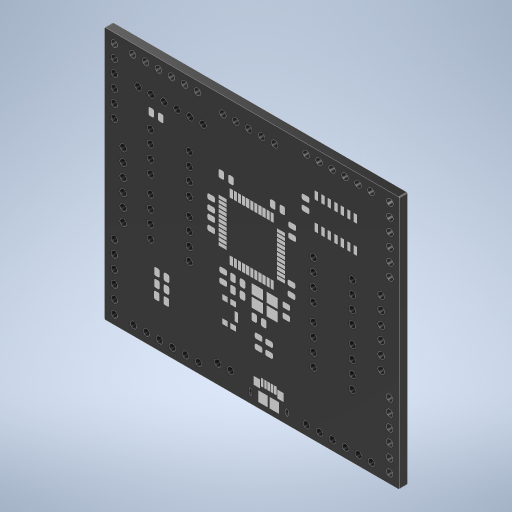
# Autodesk Inventor part: Birty.kicad_pcb
Saved by Autodesk Inventor 2023 (Build 270158000, 158)
## iProperties
Created: 2022-05-19
Part Number: Birty.kicad_pcb
Material: Generic
Document SubType Name: Modeling
Designer: Jack2bs
Density: 1 g/cm^3
Appearance: Glossy - Black
Author: Jack2bs
Autodesk Inventor part; units mm, degrees
(part 1 of 3)
ref_plane "YZ Plane" through (0, 0, 0) normal (1, 0, 0) x (0, 1, 0)
ref_plane "XZ Plane" through (0, 0, 0) normal (0, 1, 0) x (-1, 0, 0)
ref_plane "XY Plane" through (0, 0, 0) normal (0, 0, 1) x (1, 0, 0)
sketch "Sketch1" plane through (0, 0, 0) normal (0, 0, 1) x (1, 0, 0)
  line L0 (84.8868, -104.3178) -> (84.8868, -153.6446)
  arc A0 (84.8868, -153.6446) -> (85.0138, -153.7716) centre (85.0138, -153.6446) ccw
  line L1 (85.0138, -153.7716) -> (142.4432, -153.7716)
  arc A1 (142.4432, -153.7716) -> (142.5702, -153.6446) centre (142.4432, -153.6446) ccw
  line L2 (142.5702, -153.6446) -> (142.5702, -104.3178)
  arc A2 (142.5702, -104.3178) -> (142.4432, -104.1908) centre (142.4432, -104.3178) ccw
  line L3 (142.4432, -104.1908) -> (85.0138, -104.1908)
  arc A3 (85.0138, -104.1908) -> (84.8868, -104.3178) centre (85.0138, -104.3178) ccw
  line L4 (120.8178, -151.3204) -> (120.8178, -152.1204)
  arc A4 (120.3678, -152.1204) -> (120.8178, -152.1204) centre (120.5928, -152.1204) ccw
  line L5 (120.3678, -152.1204) -> (120.3678, -151.3204)
  arc A5 (120.8178, -151.3204) -> (120.3678, -151.3204) centre (120.5928, -151.3204) ccw
  line L6 (113.2178, -152.1204) -> (113.2178, -151.3204)
  arc A6 (113.6678, -151.3204) -> (113.2178, -151.3204) centre (113.4428, -151.3204) ccw
  line L7 (113.6678, -151.3204) -> (113.6678, -152.1204)
  arc A7 (113.2178, -152.1204) -> (113.6678, -152.1204) centre (113.4428, -152.1204) ccw
  circle A8 centre (103.0766, -106.067) radius 0.635
  circle A9 centre (100.5366, -106.067) radius 0.635
  circle A10 centre (92.9166, -106.067) radius 0.635
  circle A11 centre (95.4566, -106.067) radius 0.635
  circle A12 centre (90.3766, -106.067) radius 0.635
  circle A13 centre (97.9966, -106.067) radius 0.635
  circle A14 centre (137.0364, -106.0162) radius 0.635
  circle A15 centre (134.4964, -106.0162) radius 0.635
  circle A16 centre (126.8764, -106.0162) radius 0.635
  circle A17 centre (129.4164, -106.0162) radius 0.635
  circle A18 centre (124.3364, -106.0162) radius 0.635
  circle A19 centre (131.9564, -106.0162) radius 0.635
  circle A20 centre (88.519, -122.8344) radius 0.6475
  circle A21 centre (88.519, -125.3744) radius 0.6475
  circle A22 centre (88.519, -127.9144) radius 0.6475
  circle A23 centre (88.519, -130.4544) radius 0.6475
  circle A24 centre (88.519, -132.9944) radius 0.6475
  circle A25 centre (88.519, -135.5344) radius 0.6475
  circle A26 centre (139.0396, -135.3312) radius 0.6475
  circle A27 centre (139.0396, -132.7912) radius 0.6475
  circle A28 centre (139.0396, -130.2512) radius 0.6475
  circle A29 centre (139.0396, -127.7112) radius 0.6475
  circle A30 centre (139.0396, -125.1712) radius 0.6475
  circle A31 centre (139.0396, -122.6312) radius 0.6475
  circle A32 centre (86.763, -106.067) radius 0.635
  circle A33 centre (86.763, -108.607) radius 0.635
  circle A34 centre (86.763, -116.227) radius 0.635
  circle A35 centre (86.763, -113.687) radius 0.635
  circle A36 centre (86.763, -118.767) radius 0.635
  circle A37 centre (86.763, -111.147) radius 0.635
  circle A38 centre (118.1862, -107.3658) radius 0.635
  circle A39 centre (113.1062, -107.3658) radius 0.635
  circle A40 centre (108.0262, -107.3658) radius 0.635
  circle A41 centre (110.5662, -107.3658) radius 0.635
  circle A42 centre (115.6462, -107.3658) radius 0.635
  circle A43 centre (86.763, -139.2648) radius 0.635
  circle A44 centre (86.763, -141.8048) radius 0.635
  circle A45 centre (86.763, -149.4248) radius 0.635
  circle A46 centre (86.763, -146.8848) radius 0.635
  circle A47 centre (86.763, -151.9648) radius 0.635
  circle A48 centre (86.763, -144.3448) radius 0.635
  circle A49 centre (107.0102, -150.1394) radius 0.6475
  circle A50 centre (109.5502, -150.1394) radius 0.6475
  circle A51 centre (140.7448, -118.6722) radius 0.635
  circle A52 centre (140.7448, -116.1322) radius 0.635
  circle A53 centre (140.7448, -108.5122) radius 0.635
  circle A54 centre (140.7448, -111.0522) radius 0.635
  circle A55 centre (140.7448, -105.9722) radius 0.635
  circle A56 centre (140.7448, -113.5922) radius 0.635
  circle A57 centre (101.5966, -111.0776) radius 0.635
  circle A58 centre (91.4366, -111.0776) radius 0.635
  circle A59 centre (93.9766, -111.0776) radius 0.635
  circle A60 centre (96.5166, -111.0776) radius 0.635
  circle A61 centre (104.1366, -111.0776) radius 0.635
  circle A62 centre (99.0566, -111.0776) radius 0.635
  circle A63 centre (140.694, -151.8954) radius 0.635
  circle A64 centre (140.694, -149.3554) radius 0.635
  circle A65 centre (140.694, -141.7354) radius 0.635
  circle A66 centre (140.694, -144.2754) radius 0.635
  circle A67 centre (140.694, -139.1954) radius 0.635
  circle A68 centre (140.694, -146.8154) radius 0.635
  circle A69 centre (90.5476, -151.8954) radius 0.635
  circle A70 centre (93.0876, -151.8954) radius 0.635
  circle A71 centre (100.7076, -151.8954) radius 0.635
  circle A72 centre (98.1676, -151.8954) radius 0.635
  circle A73 centre (103.2476, -151.8954) radius 0.635
  circle A74 centre (95.6276, -151.8954) radius 0.635
  circle A75 centre (124.4058, -151.8954) radius 0.635
  circle A76 centre (126.9458, -151.8954) radius 0.635
  circle A77 centre (134.5658, -151.8954) radius 0.635
  circle A78 centre (132.0258, -151.8954) radius 0.635
  circle A79 centre (137.1058, -151.8954) radius 0.635
  circle A80 centre (129.4858, -151.8954) radius 0.635
  circle A81 centre (93.853, -124.6632) radius 0.635
  circle A82 centre (93.853, -122.1232) radius 0.635
  circle A83 centre (93.853, -117.0432) radius 0.635
  circle A84 centre (93.853, -119.5832) radius 0.635
  circle A85 centre (101.473, -119.5832) radius 0.635
  circle A86 centre (101.473, -117.0432) radius 0.635
  circle A87 centre (101.473, -124.6632) radius 0.635
  circle A88 centre (101.473, -122.1232) radius 0.635
  circle A89 centre (133.4008, -133.8072) radius 0.635
  circle A90 centre (133.4008, -136.3472) radius 0.635
  circle A91 centre (133.4008, -141.4272) radius 0.635
  circle A92 centre (133.4008, -138.8872) radius 0.635
  circle A93 centre (125.7808, -138.8872) radius 0.635
  circle A94 centre (125.7808, -141.4272) radius 0.635
  circle A95 centre (125.7808, -133.8072) radius 0.635
  circle A96 centre (125.7808, -136.3472) radius 0.635
  circle A97 centre (93.853, -135.6868) radius 0.635
  circle A98 centre (93.853, -133.1468) radius 0.635
  circle A99 centre (93.853, -128.0668) radius 0.635
  circle A100 centre (93.853, -130.6068) radius 0.635
  circle A101 centre (101.473, -130.6068) radius 0.635
  circle A102 centre (101.473, -128.0668) radius 0.635
  circle A103 centre (101.473, -135.6868) radius 0.635
  circle A104 centre (101.473, -133.1468) radius 0.635
  circle A105 centre (133.3754, -122.809) radius 0.635
  circle A106 centre (133.3754, -125.349) radius 0.635
  circle A107 centre (133.3754, -130.429) radius 0.635
  circle A108 centre (133.3754, -127.889) radius 0.635
  circle A109 centre (125.7554, -127.889) radius 0.635
  circle A110 centre (125.7554, -130.429) radius 0.635
  circle A111 centre (125.7554, -122.809) radius 0.635
  circle A112 centre (125.7554, -125.349) radius 0.635
  constraints: 113 centre point, 16 end point, 16 point on circle
extrude "Birty.kicad_pcb_Outline" add sketch "Sketch1" along normal blind 1.6
sketch "Sketch2" plane through (0, 0, 1.6) normal (0, 0, 1) x (1, 0, 0)
  line L0 (116.7679, -152.6705) -> (115.0178, -152.6705)
  line L1 (115.0178, -152.6705) -> (115.0178, -150.7703)
  line L2 (115.0178, -150.7703) -> (116.7679, -150.7703)
  line L3 (116.7679, -150.7703) -> (116.7679, -152.6705)
  line L4 (119.0178, -152.6705) -> (117.2677, -152.6705)
  line L5 (117.2677, -152.6705) -> (117.2677, -150.7703)
  line L6 (117.2677, -150.7703) -> (119.0178, -150.7703)
  line L7 (119.0178, -150.7703) -> (119.0178, -152.6705)
  line L8 (115.2728, -150.2153) -> (114.1227, -150.2153)
  line L9 (114.1227, -150.2153) -> (114.1227, -148.7655)
  line L10 (114.1227, -148.7655) -> (115.2728, -148.7655)
  line L11 (115.2728, -148.7655) -> (115.2728, -150.2153)
  line L12 (119.9129, -150.2153) -> (118.7628, -150.2153)
  line L13 (118.7628, -150.2153) -> (118.7628, -148.7655)
  line L14 (118.7628, -148.7655) -> (119.9129, -148.7655)
  line L15 (119.9129, -148.7655) -> (119.9129, -150.2153)
  line L16 (117.2177, -149.7703) -> (116.8179, -149.7703)
  line L17 (116.8179, -149.7703) -> (116.8179, -148.3703)
  line L18 (116.8179, -148.3703) -> (117.2177, -148.3703)
  line L19 (117.2177, -148.3703) -> (117.2177, -149.7703)
  line L20 (117.8677, -149.7703) -> (117.4679, -149.7703)
  line L21 (117.4679, -149.7703) -> (117.4679, -148.3703)
  line L22 (117.4679, -148.3703) -> (117.8677, -148.3703)
  line L23 (117.8677, -148.3703) -> (117.8677, -149.7703)
  line L24 (118.5179, -149.7703) -> (118.1179, -149.7703)
  line L25 (118.1179, -149.7703) -> (118.1179, -148.3703)
  line L26 (118.1179, -148.3703) -> (118.5179, -148.3703)
  line L27 (118.5179, -148.3703) -> (118.5179, -149.7703)
  line L28 (115.9177, -149.7703) -> (115.5177, -149.7703)
  line L29 (115.5177, -149.7703) -> (115.5177, -148.3703)
  line L30 (115.5177, -148.3703) -> (115.9177, -148.3703)
  line L31 (115.9177, -148.3703) -> (115.9177, -149.7703)
  line L32 (116.5677, -149.7703) -> (116.1679, -149.7703)
  line L33 (116.1679, -149.7703) -> (116.1679, -148.3703)
  line L34 (116.1679, -148.3703) -> (116.5677, -148.3703)
  line L35 (116.5677, -148.3703) -> (116.5677, -149.7703)
  line L36 (97.2663, -143.9832) -> (97.312, -143.9969)
  line L37 (97.312, -143.9969) -> (97.3541, -144.0195)
  line L38 (97.3541, -144.0195) -> (97.391, -144.0497)
  line L39 (97.391, -144.0497) -> (97.4214, -144.0868)
  line L40 (97.4214, -144.0868) -> (97.4438, -144.1287)
  line L41 (97.4438, -144.1287) -> (97.4578, -144.1747)
  line L42 (97.4578, -144.1747) -> (97.4623, -144.2222)
  line L43 (97.4623, -144.2222) -> (97.4623, -145.1346)
  line L44 (97.4623, -145.1346) -> (97.4578, -145.1821)
  line L45 (97.4578, -145.1821) -> (97.4438, -145.2278)
  line L46 (97.4438, -145.2278) -> (97.4214, -145.27)
  line L47 (97.4214, -145.27) -> (97.391, -145.3071)
  line L48 (97.391, -145.3071) -> (97.3541, -145.3373)
  line L49 (97.3541, -145.3373) -> (97.312, -145.3599)
  line L50 (97.312, -145.3599) -> (97.2663, -145.3736)
  line L51 (97.2663, -145.3736) -> (97.2188, -145.3784)
  line L52 (97.2188, -145.3784) -> (96.7311, -145.3784)
  line L53 (96.7311, -145.3784) -> (96.6836, -145.3736)
  line L54 (96.6836, -145.3736) -> (96.6379, -145.3599)
  line L55 (96.6379, -145.3599) -> (96.5957, -145.3373)
  line L56 (96.5957, -145.3373) -> (96.5589, -145.3071)
  line L57 (96.5589, -145.3071) -> (96.5284, -145.27)
  line L58 (96.5284, -145.27) -> (96.506, -145.2278)
  line L59 (96.506, -145.2278) -> (96.4921, -145.1821)
  line L60 (96.4921, -145.1821) -> (96.4875, -145.1346)
  line L61 (96.4875, -145.1346) -> (96.4875, -144.2222)
  line L62 (96.4875, -144.2222) -> (96.4921, -144.1747)
  line L63 (96.4921, -144.1747) -> (96.506, -144.1287)
  line L64 (96.506, -144.1287) -> (96.5284, -144.0868)
  line L65 (96.5284, -144.0868) -> (96.5589, -144.0497)
  line L66 (96.5589, -144.0497) -> (96.5957, -144.0195)
  line L67 (96.5957, -144.0195) -> (96.6379, -143.9969)
  line L68 (96.6379, -143.9969) -> (96.6836, -143.9832)
  line L69 (96.6836, -143.9832) -> (96.7311, -143.9784)
  line L70 (96.7311, -143.9784) -> (97.2188, -143.9784)
  line L71 (97.2188, -143.9784) -> (97.2663, -143.9832)
  line L72 (95.3912, -143.9832) -> (95.4369, -143.9969)
  line L73 (95.4369, -143.9969) -> (95.4791, -144.0195)
  line L74 (95.4791, -144.0195) -> (95.5159, -144.0497)
  line L75 (95.5159, -144.0497) -> (95.5464, -144.0868)
  line L76 (95.5464, -144.0868) -> (95.5688, -144.1287)
  line L77 (95.5688, -144.1287) -> (95.5827, -144.1747)
  line L78 (95.5827, -144.1747) -> (95.5873, -144.2222)
  line L79 (95.5873, -144.2222) -> (95.5873, -145.1346)
  line L80 (95.5873, -145.1346) -> (95.5827, -145.1821)
  line L81 (95.5827, -145.1821) -> (95.5688, -145.2278)
  line L82 (95.5688, -145.2278) -> (95.5464, -145.27)
  line L83 (95.5464, -145.27) -> (95.5159, -145.3071)
  line L84 (95.5159, -145.3071) -> (95.4791, -145.3373)
  line L85 (95.4791, -145.3373) -> (95.4369, -145.3599)
  line L86 (95.4369, -145.3599) -> (95.3912, -145.3736)
  line L87 (95.3912, -145.3736) -> (95.3437, -145.3784)
  line L88 (95.3437, -145.3784) -> (94.856, -145.3784)
  line L89 (94.856, -145.3784) -> (94.8085, -145.3736)
  line L90 (94.8085, -145.3736) -> (94.7628, -145.3599)
  line L91 (94.7628, -145.3599) -> (94.7207, -145.3373)
  line L92 (94.7207, -145.3373) -> (94.6838, -145.3071)
  line L93 (94.6838, -145.3071) -> (94.6534, -145.27)
  line L94 (94.6534, -145.27) -> (94.631, -145.2278)
  line L95 (94.631, -145.2278) -> (94.617, -145.1821)
  line L96 (94.617, -145.1821) -> (94.6125, -145.1346)
  line L97 (94.6125, -145.1346) -> (94.6125, -144.2222)
  line L98 (94.6125, -144.2222) -> (94.617, -144.1747)
  line L99 (94.617, -144.1747) -> (94.631, -144.1287)
  line L100 (94.631, -144.1287) -> (94.6534, -144.0868)
  line L101 (94.6534, -144.0868) -> (94.6838, -144.0497)
  line L102 (94.6838, -144.0497) -> (94.7207, -144.0195)
  line L103 (94.7207, -144.0195) -> (94.7628, -143.9969)
  line L104 (94.7628, -143.9969) -> (94.8085, -143.9832)
  line L105 (94.8085, -143.9832) -> (94.856, -143.9784)
  line L106 (94.856, -143.9784) -> (95.3437, -143.9784)
  line L107 (95.3437, -143.9784) -> (95.3912, -143.9832)
  line L108 (117.5977, -143.1011) -> (117.6437, -143.115)
  line L109 (117.6437, -143.115) -> (117.6856, -143.1374)
  line L110 (117.6856, -143.1374) -> (117.7227, -143.1679)
  line L111 (117.7227, -143.1679) -> (117.7529, -143.2047)
  line L112 (117.7529, -143.2047) -> (117.7755, -143.2469)
  line L113 (117.7755, -143.2469) -> (117.7892, -143.2926)
  line L114 (117.7892, -143.2926) -> (117.794, -143.3401)
  line L115 (117.794, -143.3401) -> (117.794, -143.8278)
  line L116 (117.794, -143.8278) -> (117.7892, -143.8753)
  line L117 (117.7892, -143.8753) -> (117.7755, -143.921)
  line L118 (117.7755, -143.921) -> (117.7529, -143.9631)
  line L119 (117.7529, -143.9631) -> (117.7227, -144)
  line L120 (117.7227, -144) -> (117.6856, -144.0304)
  line L121 (117.6856, -144.0304) -> (117.6437, -144.0528)
  line L122 (117.6437, -144.0528) -> (117.5977, -144.0668)
  line L123 (117.5977, -144.0668) -> (117.5502, -144.0713)
  line L124 (117.5502, -144.0713) -> (116.6378, -144.0713)
  line L125 (116.6378, -144.0713) -> (116.5903, -144.0668)
  line L126 (116.5903, -144.0668) -> (116.5443, -144.0528)
  line L127 (116.5443, -144.0528) -> (116.5024, -144.0304)
  line L128 (116.5024, -144.0304) -> (116.4654, -144)
  line L129 (116.4654, -144) -> (116.4351, -143.9631)
  line L130 (116.4351, -143.9631) -> (116.4125, -143.921)
  line L131 (116.4125, -143.921) -> (116.3988, -143.8753)
  line L132 (116.3988, -143.8753) -> (116.394, -143.8278)
  line L133 (116.394, -143.8278) -> (116.394, -143.3401)
  line L134 (116.394, -143.3401) -> (116.3988, -143.2926)
  line L135 (116.3988, -143.2926) -> (116.4125, -143.2469)
  line L136 (116.4125, -143.2469) -> (116.4351, -143.2047)
  line L137 (116.4351, -143.2047) -> (116.4654, -143.1679)
  line L138 (116.4654, -143.1679) -> (116.5024, -143.1374)
  line L139 (116.5024, -143.1374) -> (116.5443, -143.115)
  line L140 (116.5443, -143.115) -> (116.5903, -143.1011)
  line L141 (116.5903, -143.1011) -> (116.6378, -143.0965)
  line L142 (116.6378, -143.0965) -> (117.5502, -143.0965)
  line L143 (117.5502, -143.0965) -> (117.5977, -143.1011)
  line L144 (115.5403, -143.0779) -> (115.586, -143.0919)
  line L145 (115.586, -143.0919) -> (115.6282, -143.1143)
  line L146 (115.6282, -143.1143) -> (115.6653, -143.1447)
  line L147 (115.6653, -143.1447) -> (115.6955, -143.1816)
  line L148 (115.6955, -143.1816) -> (115.7181, -143.2237)
  line L149 (115.7181, -143.2237) -> (115.7318, -143.2695)
  line L150 (115.7318, -143.2695) -> (115.7366, -143.317)
  line L151 (115.7366, -143.317) -> (115.7366, -143.8046)
  line L152 (115.7366, -143.8046) -> (115.7318, -143.8521)
  line L153 (115.7318, -143.8521) -> (115.7181, -143.8979)
  line L154 (115.7181, -143.8979) -> (115.6955, -143.94)
  line L155 (115.6955, -143.94) -> (115.6653, -143.9769)
  line L156 (115.6653, -143.9769) -> (115.6282, -144.0073)
  line L157 (115.6282, -144.0073) -> (115.586, -144.0297)
  line L158 (115.586, -144.0297) -> (115.5403, -144.0437)
  line L159 (115.5403, -144.0437) -> (115.4928, -144.0482)
  line L160 (115.4928, -144.0482) -> (114.5804, -144.0482)
  line L161 (114.5804, -144.0482) -> (114.5329, -144.0437)
  line L162 (114.5329, -144.0437) -> (114.4872, -144.0297)
  line L163 (114.4872, -144.0297) -> (114.445, -144.0073)
  line L164 (114.445, -144.0073) -> (114.4079, -143.9769)
  line L165 (114.4079, -143.9769) -> (114.3777, -143.94)
  line L166 (114.3777, -143.94) -> (114.3551, -143.8979)
  line L167 (114.3551, -143.8979) -> (114.3414, -143.8521)
  line L168 (114.3414, -143.8521) -> (114.3366, -143.8046)
  line L169 (114.3366, -143.8046) -> (114.3366, -143.317)
  line L170 (114.3366, -143.317) -> (114.3414, -143.2695)
  line L171 (114.3414, -143.2695) -> (114.3551, -143.2237)
  line L172 (114.3551, -143.2237) -> (114.3777, -143.1816)
  line L173 (114.3777, -143.1816) -> (114.4079, -143.1447)
  line L174 (114.4079, -143.1447) -> (114.445, -143.1143)
  line L175 (114.445, -143.1143) -> (114.4872, -143.0919)
  line L176 (114.4872, -143.0919) -> (114.5329, -143.0779)
  line L177 (114.5329, -143.0779) -> (114.5804, -143.0734)
  line L178 (114.5804, -143.0734) -> (115.4928, -143.0734)
  line L179 (115.4928, -143.0734) -> (115.5403, -143.0779)
  line L180 (95.4166, -141.9512) -> (95.4623, -141.9649)
  line L181 (95.4623, -141.9649) -> (95.5045, -141.9875)
  line L182 (95.5045, -141.9875) -> (95.5413, -142.0178)
  line L183 (95.5413, -142.0178) -> (95.5718, -142.0548)
  line L184 (95.5718, -142.0548) -> (95.5942, -142.0967)
  line L185 (95.5942, -142.0967) -> (95.6081, -142.1427)
  line L186 (95.6081, -142.1427) -> (95.6127, -142.1902)
  line L187 (95.6127, -142.1902) -> (95.6127, -143.1026)
  line L188 (95.6127, -143.1026) -> (95.6081, -143.1501)
  line L189 (95.6081, -143.1501) -> (95.5942, -143.1958)
  line L190 (95.5942, -143.1958) -> (95.5718, -143.238)
  line L191 (95.5718, -143.238) -> (95.5413, -143.275)
  line L192 (95.5413, -143.275) -> (95.5045, -143.3053)
  line L193 (95.5045, -143.3053) -> (95.4623, -143.3279)
  line L194 (95.4623, -143.3279) -> (95.4166, -143.3416)
  line L195 (95.4166, -143.3416) -> (95.3691, -143.3464)
  line L196 (95.3691, -143.3464) -> (94.8814, -143.3464)
  line L197 (94.8814, -143.3464) -> (94.8339, -143.3416)
  line L198 (94.8339, -143.3416) -> (94.7882, -143.3279)
  line L199 (94.7882, -143.3279) -> (94.7461, -143.3053)
  line L200 (94.7461, -143.3053) -> (94.7092, -143.275)
  line L201 (94.7092, -143.275) -> (94.6788, -143.238)
  line L202 (94.6788, -143.238) -> (94.6564, -143.1958)
  line L203 (94.6564, -143.1958) -> (94.6424, -143.1501)
  line L204 (94.6424, -143.1501) -> (94.6379, -143.1026)
  line L205 (94.6379, -143.1026) -> (94.6379, -142.1902)
  line L206 (94.6379, -142.1902) -> (94.6424, -142.1427)
  line L207 (94.6424, -142.1427) -> (94.6564, -142.0967)
  line L208 (94.6564, -142.0967) -> (94.6788, -142.0548)
  line L209 (94.6788, -142.0548) -> (94.7092, -142.0178)
  line L210 (94.7092, -142.0178) -> (94.7461, -141.9875)
  line L211 (94.7461, -141.9875) -> (94.7882, -141.9649)
  line L212 (94.7882, -141.9649) -> (94.8339, -141.9512)
  line L213 (94.8339, -141.9512) -> (94.8814, -141.9464)
  line L214 (94.8814, -141.9464) -> (95.3691, -141.9464)
  line L215 (95.3691, -141.9464) -> (95.4166, -141.9512)
  line L216 (97.2917, -141.9512) -> (97.3374, -141.9649)
  line L217 (97.3374, -141.9649) -> (97.3795, -141.9875)
  line L218 (97.3795, -141.9875) -> (97.4164, -142.0178)
  line L219 (97.4164, -142.0178) -> (97.4468, -142.0548)
  line L220 (97.4468, -142.0548) -> (97.4692, -142.0967)
  line L221 (97.4692, -142.0967) -> (97.4832, -142.1427)
  line L222 (97.4832, -142.1427) -> (97.4877, -142.1902)
  line L223 (97.4877, -142.1902) -> (97.4877, -143.1026)
  line L224 (97.4877, -143.1026) -> (97.4832, -143.1501)
  line L225 (97.4832, -143.1501) -> (97.4692, -143.1958)
  line L226 (97.4692, -143.1958) -> (97.4468, -143.238)
  line L227 (97.4468, -143.238) -> (97.4164, -143.275)
  line L228 (97.4164, -143.275) -> (97.3795, -143.3053)
  line L229 (97.3795, -143.3053) -> (97.3374, -143.3279)
  line L230 (97.3374, -143.3279) -> (97.2917, -143.3416)
  line L231 (97.2917, -143.3416) -> (97.2442, -143.3464)
  line L232 (97.2442, -143.3464) -> (96.7565, -143.3464)
  line L233 (96.7565, -143.3464) -> (96.709, -143.3416)
  line L234 (96.709, -143.3416) -> (96.6633, -143.3279)
  line L235 (96.6633, -143.3279) -> (96.6211, -143.3053)
  line L236 (96.6211, -143.3053) -> (96.5843, -143.275)
  line L237 (96.5843, -143.275) -> (96.5538, -143.238)
  line L238 (96.5538, -143.238) -> (96.5314, -143.1958)
  line L239 (96.5314, -143.1958) -> (96.5175, -143.1501)
  line L240 (96.5175, -143.1501) -> (96.5129, -143.1026)
  line L241 (96.5129, -143.1026) -> (96.5129, -142.1902)
  line L242 (96.5129, -142.1902) -> (96.5175, -142.1427)
  line L243 (96.5175, -142.1427) -> (96.5314, -142.0967)
  line L244 (96.5314, -142.0967) -> (96.5538, -142.0548)
  line L245 (96.5538, -142.0548) -> (96.5843, -142.0178)
  line L246 (96.5843, -142.0178) -> (96.6211, -141.9875)
  line L247 (96.6211, -141.9875) -> (96.6633, -141.9649)
  line L248 (96.6633, -141.9649) -> (96.709, -141.9512)
  line L249 (96.709, -141.9512) -> (96.7565, -141.9464)
  line L250 (96.7565, -141.9464) -> (97.2442, -141.9464)
  line L251 (97.2442, -141.9464) -> (97.2917, -141.9512)
  line L252 (108.9454, -142.9621) -> (107.9454, -142.9621)
  line L253 (107.9454, -142.9621) -> (107.9454, -142.0619)
  line L254 (107.9454, -142.0619) -> (108.9454, -142.0619)
  line L255 (108.9454, -142.0619) -> (108.9454, -142.9621)
  line L256 (110.5454, -142.9621) -> (109.5454, -142.9621)
  line L257 (109.5454, -142.9621) -> (109.5454, -142.0619)
  line L258 (109.5454, -142.0619) -> (110.5454, -142.0619)
  line L259 (110.5454, -142.0619) -> (110.5454, -142.9621)
  line L260 (117.5977, -141.226) -> (117.6437, -141.24)
  line L261 (117.6437, -141.24) -> (117.6856, -141.2624)
  line L262 (117.6856, -141.2624) -> (117.7227, -141.2928)
  line L263 (117.7227, -141.2928) -> (117.7529, -141.3297)
  line L264 (117.7529, -141.3297) -> (117.7755, -141.3718)
  line L265 (117.7755, -141.3718) -> (117.7892, -141.4175)
  line L266 (117.7892, -141.4175) -> (117.794, -141.465)
  line L267 (117.794, -141.465) -> (117.794, -141.9527)
  line L268 (117.794, -141.9527) -> (117.7892, -142.0002)
  line L269 (117.7892, -142.0002) -> (117.7755, -142.0459)
  line L270 (117.7755, -142.0459) -> (117.7529, -142.0881)
  line L271 (117.7529, -142.0881) -> (117.7227, -142.1249)
  line L272 (117.7227, -142.1249) -> (117.6856, -142.1554)
  line L273 (117.6856, -142.1554) -> (117.6437, -142.1778)
  line L274 (117.6437, -142.1778) -> (117.5977, -142.1917)
  line L275 (117.5977, -142.1917) -> (117.5502, -142.1963)
  line L276 (117.5502, -142.1963) -> (116.6378, -142.1963)
  line L277 (116.6378, -142.1963) -> (116.5903, -142.1917)
  line L278 (116.5903, -142.1917) -> (116.5443, -142.1778)
  line L279 (116.5443, -142.1778) -> (116.5024, -142.1554)
  line L280 (116.5024, -142.1554) -> (116.4654, -142.1249)
  line L281 (116.4654, -142.1249) -> (116.4351, -142.0881)
  line L282 (116.4351, -142.0881) -> (116.4125, -142.0459)
  line L283 (116.4125, -142.0459) -> (116.3988, -142.0002)
  line L284 (116.3988, -142.0002) -> (116.394, -141.9527)
  line L285 (116.394, -141.9527) -> (116.394, -141.465)
  line L286 (116.394, -141.465) -> (116.3988, -141.4175)
  line L287 (116.3988, -141.4175) -> (116.4125, -141.3718)
  line L288 (116.4125, -141.3718) -> (116.4351, -141.3297)
  line L289 (116.4351, -141.3297) -> (116.4654, -141.2928)
  line L290 (116.4654, -141.2928) -> (116.5024, -141.2624)
  line L291 (116.5024, -141.2624) -> (116.5443, -141.24)
  line L292 (116.5443, -141.24) -> (116.5903, -141.226)
  line L293 (116.5903, -141.226) -> (116.6378, -141.2215)
  line L294 (116.6378, -141.2215) -> (117.5502, -141.2215)
  line L295 (117.5502, -141.2215) -> (117.5977, -141.226)
  line L296 (115.5403, -141.2029) -> (115.586, -141.2169)
  line L297 (115.586, -141.2169) -> (115.6282, -141.2395)
  line L298 (115.6282, -141.2395) -> (115.6653, -141.2697)
  line L299 (115.6653, -141.2697) -> (115.6955, -141.3066)
  line L300 (115.6955, -141.3066) -> (115.7181, -141.3487)
  line L301 (115.7181, -141.3487) -> (115.7318, -141.3944)
  line L302 (115.7318, -141.3944) -> (115.7366, -141.4419)
  line L303 (115.7366, -141.4419) -> (115.7366, -141.9296)
  line L304 (115.7366, -141.9296) -> (115.7318, -141.9771)
  line L305 (115.7318, -141.9771) -> (115.7181, -142.0228)
  line L306 (115.7181, -142.0228) -> (115.6955, -142.065)
  line L307 (115.6955, -142.065) -> (115.6653, -142.1018)
  line L308 (115.6653, -142.1018) -> (115.6282, -142.1323)
  line L309 (115.6282, -142.1323) -> (115.586, -142.1547)
  line L310 (115.586, -142.1547) -> (115.5403, -142.1686)
  line L311 (115.5403, -142.1686) -> (115.4928, -142.1732)
  line L312 (115.4928, -142.1732) -> (114.5804, -142.1732)
  line L313 (114.5804, -142.1732) -> (114.5329, -142.1686)
  line L314 (114.5329, -142.1686) -> (114.4872, -142.1547)
  line L315 (114.4872, -142.1547) -> (114.445, -142.1323)
  line L316 (114.445, -142.1323) -> (114.4079, -142.1018)
  line L317 (114.4079, -142.1018) -> (114.3777, -142.065)
  line L318 (114.3777, -142.065) -> (114.3551, -142.0228)
  line L319 (114.3551, -142.0228) -> (114.3414, -141.9771)
  line L320 (114.3414, -141.9771) -> (114.3366, -141.9296)
  line L321 (114.3366, -141.9296) -> (114.3366, -141.4419)
  line L322 (114.3366, -141.4419) -> (114.3414, -141.3944)
  line L323 (114.3414, -141.3944) -> (114.3551, -141.3487)
  line L324 (114.3551, -141.3487) -> (114.3777, -141.3066)
  line L325 (114.3777, -141.3066) -> (114.4079, -141.2697)
  line L326 (114.4079, -141.2697) -> (114.445, -141.2395)
  line L327 (114.445, -141.2395) -> (114.4872, -141.2169)
  line L328 (114.4872, -141.2169) -> (114.5329, -141.2029)
  line L329 (114.5329, -141.2029) -> (114.5804, -141.1983)
  line L330 (114.5804, -141.1983) -> (115.4928, -141.1983)
  line L331 (115.4928, -141.1983) -> (115.5403, -141.2029)
  line L332 (95.4166, -139.9446) -> (95.4623, -139.9583)
  line L333 (95.4623, -139.9583) -> (95.5045, -139.9809)
  line L334 (95.5045, -139.9809) -> (95.5413, -140.0112)
  line L335 (95.5413, -140.0112) -> (95.5718, -140.0482)
  line L336 (95.5718, -140.0482) -> (95.5942, -140.0904)
  line L337 (95.5942, -140.0904) -> (95.6081, -140.1361)
  line L338 (95.6081, -140.1361) -> (95.6127, -140.1836)
  line L339 (95.6127, -140.1836) -> (95.6127, -141.096)
  line L340 (95.6127, -141.096) -> (95.6081, -141.1435)
  line L341 (95.6081, -141.1435) -> (95.5942, -141.1892)
  line L342 (95.5942, -141.1892) -> (95.5718, -141.2314)
  line L343 (95.5718, -141.2314) -> (95.5413, -141.2685)
  line L344 (95.5413, -141.2685) -> (95.5045, -141.2987)
  line L345 (95.5045, -141.2987) -> (95.4623, -141.3213)
  line L346 (95.4623, -141.3213) -> (95.4166, -141.335)
  line L347 (95.4166, -141.335) -> (95.3691, -141.3398)
  line L348 (95.3691, -141.3398) -> (94.8814, -141.3398)
  line L349 (94.8814, -141.3398) -> (94.8339, -141.335)
  line L350 (94.8339, -141.335) -> (94.7882, -141.3213)
  line L351 (94.7882, -141.3213) -> (94.7461, -141.2987)
  line L352 (94.7461, -141.2987) -> (94.7092, -141.2685)
  line L353 (94.7092, -141.2685) -> (94.6788, -141.2314)
  line L354 (94.6788, -141.2314) -> (94.6564, -141.1892)
  line L355 (94.6564, -141.1892) -> (94.6424, -141.1435)
  line L356 (94.6424, -141.1435) -> (94.6379, -141.096)
  line L357 (94.6379, -141.096) -> (94.6379, -140.1836)
  line L358 (94.6379, -140.1836) -> (94.6424, -140.1361)
  line L359 (94.6424, -140.1361) -> (94.6564, -140.0904)
  line L360 (94.6564, -140.0904) -> (94.6788, -140.0482)
  line L361 (94.6788, -140.0482) -> (94.7092, -140.0112)
  line L362 (94.7092, -140.0112) -> (94.7461, -139.9809)
  line L363 (94.7461, -139.9809) -> (94.7882, -139.9583)
  line L364 (94.7882, -139.9583) -> (94.8339, -139.9446)
  line L365 (94.8339, -139.9446) -> (94.8814, -139.9398)
  line L366 (94.8814, -139.9398) -> (95.3691, -139.9398)
  line L367 (95.3691, -139.9398) -> (95.4166, -139.9446)
  line L368 (97.2917, -139.9446) -> (97.3374, -139.9583)
  line L369 (97.3374, -139.9583) -> (97.3795, -139.9809)
  line L370 (97.3795, -139.9809) -> (97.4164, -140.0112)
  line L371 (97.4164, -140.0112) -> (97.4468, -140.0482)
  line L372 (97.4468, -140.0482) -> (97.4692, -140.0904)
  line L373 (97.4692, -140.0904) -> (97.4832, -140.1361)
  line L374 (97.4832, -140.1361) -> (97.4877, -140.1836)
  line L375 (97.4877, -140.1836) -> (97.4877, -141.096)
  line L376 (97.4877, -141.096) -> (97.4832, -141.1435)
  line L377 (97.4832, -141.1435) -> (97.4692, -141.1892)
  line L378 (97.4692, -141.1892) -> (97.4468, -141.2314)
  line L379 (97.4468, -141.2314) -> (97.4164, -141.2685)
  line L380 (97.4164, -141.2685) -> (97.3795, -141.2987)
  line L381 (97.3795, -141.2987) -> (97.3374, -141.3213)
  line L382 (97.3374, -141.3213) -> (97.2917, -141.335)
  line L383 (97.2917, -141.335) -> (97.2442, -141.3398)
  line L384 (97.2442, -141.3398) -> (96.7565, -141.3398)
  line L385 (96.7565, -141.3398) -> (96.709, -141.335)
  line L386 (96.709, -141.335) -> (96.6633, -141.3213)
  line L387 (96.6633, -141.3213) -> (96.6211, -141.2987)
  line L388 (96.6211, -141.2987) -> (96.5843, -141.2685)
  line L389 (96.5843, -141.2685) -> (96.5538, -141.2314)
  line L390 (96.5538, -141.2314) -> (96.5314, -141.1892)
  line L391 (96.5314, -141.1892) -> (96.5175, -141.1435)
  line L392 (96.5175, -141.1435) -> (96.5129, -141.096)
  line L393 (96.5129, -141.096) -> (96.5129, -140.1836)
  line L394 (96.5129, -140.1836) -> (96.5175, -140.1361)
  line L395 (96.5175, -140.1361) -> (96.5314, -140.0904)
  line L396 (96.5314, -140.0904) -> (96.5538, -140.0482)
  line L397 (96.5538, -140.0482) -> (96.5843, -140.0112)
  line L398 (96.5843, -140.0112) -> (96.6211, -139.9809)
  line L399 (96.6211, -139.9809) -> (96.6633, -139.9583)
  line L400 (96.6633, -139.9583) -> (96.709, -139.9446)
  line L401 (96.709, -139.9446) -> (96.7565, -139.9398)
  line L402 (96.7565, -139.9398) -> (97.2442, -139.9398)
  line L403 (97.2442, -139.9398) -> (97.2917, -139.9446)
  line L404 (110.9454, -141.3119) -> (110.3955, -141.3119)
  line L405 (110.3955, -141.3119) -> (110.3955, -139.6121)
  line L406 (110.3955, -139.6121) -> (110.9454, -139.6121)
  line L407 (110.9454, -139.6121) -> (110.9454, -141.3119)
  line L408 (116.3439, -138.1158) -> (116.3897, -138.1295)
  line L409 (116.3897, -138.1295) -> (116.4318, -138.1521)
  line L410 (116.4318, -138.1521) -> (116.4687, -138.1823)
  line L411 (116.4687, -138.1823) -> (116.4991, -138.2194)
  line L412 (116.4991, -138.2194) -> (116.5215, -138.2616)
  line L413 (116.5215, -138.2616) -> (116.5355, -138.3073)
  line L414 (116.5355, -138.3073) -> (116.54, -138.3548)
  line L415 (116.54, -138.3548) -> (116.54, -139.2672)
  line L416 (116.54, -139.2672) -> (116.5355, -139.3147)
  line L417 (116.5355, -139.3147) -> (116.5215, -139.3604)
  line L418 (116.5215, -139.3604) -> (116.4991, -139.4026)
  line L419 (116.4991, -139.4026) -> (116.4687, -139.4397)
  line L420 (116.4687, -139.4397) -> (116.4318, -139.4699)
  line L421 (116.4318, -139.4699) -> (116.3897, -139.4925)
  line L422 (116.3897, -139.4925) -> (116.3439, -139.5062)
  line L423 (116.3439, -139.5062) -> (116.2964, -139.511)
  line L424 (116.2964, -139.511) -> (115.8088, -139.511)
  line L425 (115.8088, -139.511) -> (115.7613, -139.5062)
  line L426 (115.7613, -139.5062) -> (115.7155, -139.4925)
  line L427 (115.7155, -139.4925) -> (115.6734, -139.4699)
  line L428 (115.6734, -139.4699) -> (115.6365, -139.4397)
  line L429 (115.6365, -139.4397) -> (115.6061, -139.4026)
  line L430 (115.6061, -139.4026) -> (115.5837, -139.3604)
  line L431 (115.5837, -139.3604) -> (115.5697, -139.3147)
  line L432 (115.5697, -139.3147) -> (115.5652, -139.2672)
  line L433 (115.5652, -139.2672) -> (115.5652, -138.3548)
  line L434 (115.5652, -138.3548) -> (115.5697, -138.3073)
  line L435 (115.5697, -138.3073) -> (115.5837, -138.2616)
  line L436 (115.5837, -138.2616) -> (115.6061, -138.2194)
  line L437 (115.6061, -138.2194) -> (115.6365, -138.1823)
  line L438 (115.6365, -138.1823) -> (115.6734, -138.1521)
  line L439 (115.6734, -138.1521) -> (115.7155, -138.1295)
  line L440 (115.7155, -138.1295) -> (115.7613, -138.1158)
  line L441 (115.7613, -138.1158) -> (115.8088, -138.111)
  line L442 (115.8088, -138.111) -> (116.2964, -138.111)
  line L443 (116.2964, -138.111) -> (116.3439, -138.1158)
  line L444 (114.4689, -138.1158) -> (114.5146, -138.1295)
  line L445 (114.5146, -138.1295) -> (114.5568, -138.1521)
  line L446 (114.5568, -138.1521) -> (114.5936, -138.1823)
  line L447 (114.5936, -138.1823) -> (114.6241, -138.2194)
  line L448 (114.6241, -138.2194) -> (114.6465, -138.2616)
  line L449 (114.6465, -138.2616) -> (114.6604, -138.3073)
  line L450 (114.6604, -138.3073) -> (114.665, -138.3548)
  line L451 (114.665, -138.3548) -> (114.665, -139.2672)
  line L452 (114.665, -139.2672) -> (114.6604, -139.3147)
  line L453 (114.6604, -139.3147) -> (114.6465, -139.3604)
  line L454 (114.6465, -139.3604) -> (114.6241, -139.4026)
  line L455 (114.6241, -139.4026) -> (114.5936, -139.4397)
  line L456 (114.5936, -139.4397) -> (114.5568, -139.4699)
  line L457 (114.5568, -139.4699) -> (114.5146, -139.4925)
  line L458 (114.5146, -139.4925) -> (114.4689, -139.5062)
  line L459 (114.4689, -139.5062) -> (114.4214, -139.511)
  line L460 (114.4214, -139.511) -> (113.9337, -139.511)
  line L461 (113.9337, -139.511) -> (113.8862, -139.5062)
  line L462 (113.8862, -139.5062) -> (113.8405, -139.4925)
  line L463 (113.8405, -139.4925) -> (113.7983, -139.4699)
  line L464 (113.7983, -139.4699) -> (113.7615, -139.4397)
  line L465 (113.7615, -139.4397) -> (113.7313, -139.4026)
  line L466 (113.7313, -139.4026) -> (113.7087, -139.3604)
  line L467 (113.7087, -139.3604) -> (113.6947, -139.3147)
  line L468 (113.6947, -139.3147) -> (113.6901, -139.2672)
  line L469 (113.6901, -139.2672) -> (113.6901, -138.3548)
  line L470 (113.6901, -138.3548) -> (113.6947, -138.3073)
  line L471 (113.6947, -138.3073) -> (113.7087, -138.2616)
  line L472 (113.7087, -138.2616) -> (113.7313, -138.2194)
  line L473 (113.7313, -138.2194) -> (113.7615, -138.1823)
  line L474 (113.7615, -138.1823) -> (113.7983, -138.1521)
  line L475 (113.7983, -138.1521) -> (113.8405, -138.1295)
  line L476 (113.8405, -138.1295) -> (113.8862, -138.1158)
  line L477 (113.8862, -138.1158) -> (113.9337, -138.111)
  line L478 (113.9337, -138.111) -> (114.4214, -138.111)
  line L479 (114.4214, -138.111) -> (114.4689, -138.1158)
  line L480 (108.9454, -138.8621) -> (107.9454, -138.8621)
  line L481 (107.9454, -138.8621) -> (107.9454, -137.9619)
  line L482 (107.9454, -137.9619) -> (108.9454, -137.9619)
  line L483 (108.9454, -137.9619) -> (108.9454, -138.8621)
  line L484 (110.5454, -138.8621) -> (109.5454, -138.8621)
  line L485 (109.5454, -138.8621) -> (109.5454, -137.9619)
  line L486 (109.5454, -137.9619) -> (110.5454, -137.9619)
  line L487 (110.5454, -137.9619) -> (110.5454, -138.8621)
  line L488 (115.8304, -137.3304) -> (113.7303, -137.3304)
  line L489 (113.7303, -137.3304) -> (113.7303, -135.5303)
  line L490 (113.7303, -135.5303) -> (115.8304, -135.5303)
  line L491 (115.8304, -135.5303) -> (115.8304, -137.3304)
  line L492 (118.7305, -137.3304) -> (116.6304, -137.3304)
  line L493 (116.6304, -137.3304) -> (116.6304, -135.5303)
  line L494 (116.6304, -135.5303) -> (118.7305, -135.5303)
  line L495 (118.7305, -135.5303) -> (118.7305, -137.3304)
  line L496 (112.1783, -135.525) -> (112.2241, -135.5387)
  line L497 (112.2241, -135.5387) -> (112.2662, -135.5613)
  line L498 (112.2662, -135.5613) -> (112.3031, -135.5916)
  line L499 (112.3031, -135.5916) -> (112.3335, -135.6286)
  line L500 (112.3335, -135.6286) -> (112.3559, -135.6705)
  line L501 (112.3559, -135.6705) -> (112.3699, -135.7165)
  line L502 (112.3699, -135.7165) -> (112.3744, -135.764)
  line L503 (112.3744, -135.764) -> (112.3744, -136.6764)
  line L504 (112.3744, -136.6764) -> (112.3699, -136.7239)
  line L505 (112.3699, -136.7239) -> (112.3559, -136.7699)
  line L506 (112.3559, -136.7699) -> (112.3335, -136.8118)
  line L507 (112.3335, -136.8118) -> (112.3031, -136.8488)
  line L508 (112.3031, -136.8488) -> (112.2662, -136.8791)
  line L509 (112.2662, -136.8791) -> (112.2241, -136.9017)
  line L510 (112.2241, -136.9017) -> (112.1783, -136.9154)
  line L511 (112.1783, -136.9154) -> (112.1308, -136.9202)
  line L512 (112.1308, -136.9202) -> (111.6432, -136.9202)
  line L513 (111.6432, -136.9202) -> (111.5957, -136.9154)
  line L514 (111.5957, -136.9154) -> (111.5499, -136.9017)
  line L515 (111.5499, -136.9017) -> (111.5078, -136.8791)
  line L516 (111.5078, -136.8791) -> (111.4709, -136.8488)
  line L517 (111.4709, -136.8488) -> (111.4405, -136.8118)
  line L518 (111.4405, -136.8118) -> (111.4181, -136.7699)
  line L519 (111.4181, -136.7699) -> (111.4041, -136.7239)
  line L520 (111.4041, -136.7239) -> (111.3996, -136.6764)
  line L521 (111.3996, -136.6764) -> (111.3996, -135.764)
  line L522 (111.3996, -135.764) -> (111.4041, -135.7165)
  line L523 (111.4041, -135.7165) -> (111.4181, -135.6705)
  line L524 (111.4181, -135.6705) -> (111.4405, -135.6286)
  line L525 (111.4405, -135.6286) -> (111.4709, -135.5916)
  line L526 (111.4709, -135.5916) -> (111.5078, -135.5613)
  line L527 (111.5078, -135.5613) -> (111.5499, -135.5387)
  line L528 (111.5499, -135.5387) -> (111.5957, -135.525)
  line L529 (111.5957, -135.525) -> (111.6432, -135.5202)
  line L530 (111.6432, -135.5202) -> (112.1308, -135.5202)
  line L531 (112.1308, -135.5202) -> (112.1783, -135.525)
  line L532 (110.3033, -135.525) -> (110.349, -135.5387)
  line L533 (110.349, -135.5387) -> (110.3912, -135.5613)
  line L534 (110.3912, -135.5613) -> (110.428, -135.5916)
  line L535 (110.428, -135.5916) -> (110.4585, -135.6286)
  line L536 (110.4585, -135.6286) -> (110.4809, -135.6705)
  line L537 (110.4809, -135.6705) -> (110.4948, -135.7165)
  line L538 (110.4948, -135.7165) -> (110.4994, -135.764)
  line L539 (110.4994, -135.764) -> (110.4994, -136.6764)
  line L540 (110.4994, -136.6764) -> (110.4948, -136.7239)
  line L541 (110.4948, -136.7239) -> (110.4809, -136.7699)
  line L542 (110.4809, -136.7699) -> (110.4585, -136.8118)
  line L543 (110.4585, -136.8118) -> (110.428, -136.8488)
  line L544 (110.428, -136.8488) -> (110.3912, -136.8791)
  line L545 (110.3912, -136.8791) -> (110.349, -136.9017)
  line L546 (110.349, -136.9017) -> (110.3033, -136.9154)
  line L547 (110.3033, -136.9154) -> (110.2558, -136.9202)
  line L548 (110.2558, -136.9202) -> (109.7681, -136.9202)
  line L549 (109.7681, -136.9202) -> (109.7206, -136.9154)
  line L550 (109.7206, -136.9154) -> (109.6749, -136.9017)
  line L551 (109.6749, -136.9017) -> (109.6328, -136.8791)
  line L552 (109.6328, -136.8791) -> (109.5959, -136.8488)
  line L553 (109.5959, -136.8488) -> (109.5657, -136.8118)
  line L554 (109.5657, -136.8118) -> (109.5431, -136.7699)
  line L555 (109.5431, -136.7699) -> (109.5291, -136.7239)
  line L556 (109.5291, -136.7239) -> (109.5245, -136.6764)
  line L557 (109.5245, -136.6764) -> (109.5245, -135.764)
  line L558 (109.5245, -135.764) -> (109.5291, -135.7165)
  line L559 (109.5291, -135.7165) -> (109.5431, -135.6705)
  line L560 (109.5431, -135.6705) -> (109.5657, -135.6286)
  line L561 (109.5657, -135.6286) -> (109.5959, -135.5916)
  line L562 (109.5959, -135.5916) -> (109.6328, -135.5613)
  line L563 (109.6328, -135.5613) -> (109.6749, -135.5387)
  line L564 (109.6749, -135.5387) -> (109.7206, -135.525)
  line L565 (109.7206, -135.525) -> (109.7681, -135.5202)
  line L566 (109.7681, -135.5202) -> (110.2558, -135.5202)
  line L567 (110.2558, -135.5202) -> (110.3033, -135.525)
  line L568 (108.6061, -135.3541) -> (108.6521, -135.368)
  line L569 (108.6521, -135.368) -> (108.694, -135.3904)
  line L570 (108.694, -135.3904) -> (108.7311, -135.4209)
  line L571 (108.7311, -135.4209) -> (108.7613, -135.4577)
  line L572 (108.7613, -135.4577) -> (108.7839, -135.4999)
  line L573 (108.7839, -135.4999) -> (108.7976, -135.5456)
  line L574 (108.7976, -135.5456) -> (108.8024, -135.5931)
  line L575 (108.8024, -135.5931) -> (108.8024, -136.0808)
  line L576 (108.8024, -136.0808) -> (108.7976, -136.1283)
  line L577 (108.7976, -136.1283) -> (108.7839, -136.174)
  line L578 (108.7839, -136.174) -> (108.7613, -136.2161)
  line L579 (108.7613, -136.2161) -> (108.7311, -136.253)
  line L580 (108.7311, -136.253) -> (108.694, -136.2834)
  line L581 (108.694, -136.2834) -> (108.6521, -136.3058)
  line L582 (108.6521, -136.3058) -> (108.6061, -136.3198)
  line L583 (108.6061, -136.3198) -> (108.5586, -136.3243)
  line L584 (108.5586, -136.3243) -> (107.6462, -136.3243)
  line L585 (107.6462, -136.3243) -> (107.5987, -136.3198)
  line L586 (107.5987, -136.3198) -> (107.5527, -136.3058)
  line L587 (107.5527, -136.3058) -> (107.5108, -136.2834)
  line L588 (107.5108, -136.2834) -> (107.4737, -136.253)
  line L589 (107.4737, -136.253) -> (107.4435, -136.2161)
  line L590 (107.4435, -136.2161) -> (107.4209, -136.174)
  line L591 (107.4209, -136.174) -> (107.4072, -136.1283)
  line L592 (107.4072, -136.1283) -> (107.4024, -136.0808)
  line L593 (107.4024, -136.0808) -> (107.4024, -135.5931)
  line L594 (107.4024, -135.5931) -> (107.4072, -135.5456)
  line L595 (107.4072, -135.5456) -> (107.4209, -135.4999)
  line L596 (107.4209, -135.4999) -> (107.4435, -135.4577)
  line L597 (107.4435, -135.4577) -> (107.4737, -135.4209)
  line L598 (107.4737, -135.4209) -> (107.5108, -135.3904)
  line L599 (107.5108, -135.3904) -> (107.5527, -135.368)
  line L600 (107.5527, -135.368) -> (107.5987, -135.3541)
  line L601 (107.5987, -135.3541) -> (107.6462, -135.3495)
  line L602 (107.6462, -135.3495) -> (108.5586, -135.3495)
  line L603 (108.5586, -135.3495) -> (108.6061, -135.3541)
  line L604 (120.9759, -135.1255) -> (121.0219, -135.1394)
  line L605 (121.0219, -135.1394) -> (121.0638, -135.1618)
  line L606 (121.0638, -135.1618) -> (121.1009, -135.1923)
  line L607 (121.1009, -135.1923) -> (121.1311, -135.2291)
  line L608 (121.1311, -135.2291) -> (121.1537, -135.2713)
  line L609 (121.1537, -135.2713) -> (121.1674, -135.317)
  line L610 (121.1674, -135.317) -> (121.1722, -135.3645)
  line L611 (121.1722, -135.3645) -> (121.1722, -135.8522)
  line L612 (121.1722, -135.8522) -> (121.1674, -135.8997)
  line L613 (121.1674, -135.8997) -> (121.1537, -135.9454)
  line L614 (121.1537, -135.9454) -> (121.1311, -135.9875)
  line L615 (121.1311, -135.9875) -> (121.1009, -136.0244)
  line L616 (121.1009, -136.0244) -> (121.0638, -136.0548)
  line L617 (121.0638, -136.0548) -> (121.0219, -136.0772)
  line L618 (121.0219, -136.0772) -> (120.9759, -136.0912)
  line L619 (120.9759, -136.0912) -> (120.9284, -136.0957)
  line L620 (120.9284, -136.0957) -> (120.016, -136.0957)
  line L621 (120.016, -136.0957) -> (119.9685, -136.0912)
  line L622 (119.9685, -136.0912) -> (119.9225, -136.0772)
  line L623 (119.9225, -136.0772) -> (119.8806, -136.0548)
  line L624 (119.8806, -136.0548) -> (119.8436, -136.0244)
  line L625 (119.8436, -136.0244) -> (119.8133, -135.9875)
  line L626 (119.8133, -135.9875) -> (119.7907, -135.9454)
  line L627 (119.7907, -135.9454) -> (119.777, -135.8997)
  line L628 (119.777, -135.8997) -> (119.7722, -135.8522)
  line L629 (119.7722, -135.8522) -> (119.7722, -135.3645)
  line L630 (119.7722, -135.3645) -> (119.777, -135.317)
  line L631 (119.777, -135.317) -> (119.7907, -135.2713)
  line L632 (119.7907, -135.2713) -> (119.8133, -135.2291)
  line L633 (119.8133, -135.2291) -> (119.8436, -135.1923)
  line L634 (119.8436, -135.1923) -> (119.8806, -135.1618)
  line L635 (119.8806, -135.1618) -> (119.9225, -135.1394)
  line L636 (119.9225, -135.1394) -> (119.9685, -135.1255)
  line L637 (119.9685, -135.1255) -> (120.016, -135.1209)
  line L638 (120.016, -135.1209) -> (120.9284, -135.1209)
  line L639 (120.9284, -135.1209) -> (120.9759, -135.1255)
  line L640 (118.7305, -135.0305) -> (116.6304, -135.0305)
  line L641 (116.6304, -135.0305) -> (116.6304, -133.2304)
  line L642 (116.6304, -133.2304) -> (118.7305, -133.2304)
  line L643 (118.7305, -133.2304) -> (118.7305, -135.0305)
  line L644 (115.8304, -135.0305) -> (113.7303, -135.0305)
  line L645 (113.7303, -135.0305) -> (113.7303, -133.2304)
  line L646 (113.7303, -133.2304) -> (115.8304, -133.2304)
  line L647 (115.8304, -133.2304) -> (115.8304, -135.0305)
  line L648 (110.3033, -133.4676) -> (110.349, -133.4813)
  line L649 (110.349, -133.4813) -> (110.3912, -133.5039)
  line L650 (110.3912, -133.5039) -> (110.428, -133.5342)
  line L651 (110.428, -133.5342) -> (110.4585, -133.5712)
  line L652 (110.4585, -133.5712) -> (110.4809, -133.6134)
  line L653 (110.4809, -133.6134) -> (110.4948, -133.6591)
  line L654 (110.4948, -133.6591) -> (110.4994, -133.7066)
  line L655 (110.4994, -133.7066) -> (110.4994, -134.619)
  line L656 (110.4994, -134.619) -> (110.4948, -134.6665)
  line L657 (110.4948, -134.6665) -> (110.4809, -134.7122)
  line L658 (110.4809, -134.7122) -> (110.4585, -134.7544)
  line L659 (110.4585, -134.7544) -> (110.428, -134.7914)
  line L660 (110.428, -134.7914) -> (110.3912, -134.8217)
  line L661 (110.3912, -134.8217) -> (110.349, -134.8443)
  line L662 (110.349, -134.8443) -> (110.3033, -134.858)
  line L663 (110.3033, -134.858) -> (110.2558, -134.8628)
  line L664 (110.2558, -134.8628) -> (109.7681, -134.8628)
  line L665 (109.7681, -134.8628) -> (109.7206, -134.858)
  line L666 (109.7206, -134.858) -> (109.6749, -134.8443)
  line L667 (109.6749, -134.8443) -> (109.6328, -134.8217)
  line L668 (109.6328, -134.8217) -> (109.5959, -134.7914)
  line L669 (109.5959, -134.7914) -> (109.5657, -134.7544)
  line L670 (109.5657, -134.7544) -> (109.5431, -134.7122)
  line L671 (109.5431, -134.7122) -> (109.5291, -134.6665)
  line L672 (109.5291, -134.6665) -> (109.5245, -134.619)
  line L673 (109.5245, -134.619) -> (109.5245, -133.7066)
  line L674 (109.5245, -133.7066) -> (109.5291, -133.6591)
  line L675 (109.5291, -133.6591) -> (109.5431, -133.6134)
  line L676 (109.5431, -133.6134) -> (109.5657, -133.5712)
  line L677 (109.5657, -133.5712) -> (109.5959, -133.5342)
  line L678 (109.5959, -133.5342) -> (109.6328, -133.5039)
  line L679 (109.6328, -133.5039) -> (109.6749, -133.4813)
  line L680 (109.6749, -133.4813) -> (109.7206, -133.4676)
  line L681 (109.7206, -133.4676) -> (109.7681, -133.4628)
  line L682 (109.7681, -133.4628) -> (110.2558, -133.4628)
  line L683 (110.2558, -133.4628) -> (110.3033, -133.4676)
  line L684 (112.1783, -133.4676) -> (112.2241, -133.4813)
  line L685 (112.2241, -133.4813) -> (112.2662, -133.5039)
  line L686 (112.2662, -133.5039) -> (112.3031, -133.5342)
  line L687 (112.3031, -133.5342) -> (112.3335, -133.5712)
  line L688 (112.3335, -133.5712) -> (112.3559, -133.6134)
  line L689 (112.3559, -133.6134) -> (112.3699, -133.6591)
  line L690 (112.3699, -133.6591) -> (112.3744, -133.7066)
  line L691 (112.3744, -133.7066) -> (112.3744, -134.619)
  line L692 (112.3744, -134.619) -> (112.3699, -134.6665)
  line L693 (112.3699, -134.6665) -> (112.3559, -134.7122)
  line L694 (112.3559, -134.7122) -> (112.3335, -134.7544)
  line L695 (112.3335, -134.7544) -> (112.3031, -134.7914)
  line L696 (112.3031, -134.7914) -> (112.2662, -134.8217)
  line L697 (112.2662, -134.8217) -> (112.2241, -134.8443)
  line L698 (112.2241, -134.8443) -> (112.1783, -134.858)
  line L699 (112.1783, -134.858) -> (112.1308, -134.8628)
  line L700 (112.1308, -134.8628) -> (111.6432, -134.8628)
  line L701 (111.6432, -134.8628) -> (111.5957, -134.858)
  line L702 (111.5957, -134.858) -> (111.5499, -134.8443)
  line L703 (111.5499, -134.8443) -> (111.5078, -134.8217)
  line L704 (111.5078, -134.8217) -> (111.4709, -134.7914)
  line L705 (111.4709, -134.7914) -> (111.4405, -134.7544)
  line L706 (111.4405, -134.7544) -> (111.4181, -134.7122)
  line L707 (111.4181, -134.7122) -> (111.4041, -134.6665)
  line L708 (111.4041, -134.6665) -> (111.3996, -134.619)
  line L709 (111.3996, -134.619) -> (111.3996, -133.7066)
  line L710 (111.3996, -133.7066) -> (111.4041, -133.6591)
  line L711 (111.4041, -133.6591) -> (111.4181, -133.6134)
  line L712 (111.4181, -133.6134) -> (111.4405, -133.5712)
  line L713 (111.4405, -133.5712) -> (111.4709, -133.5342)
  line L714 (111.4709, -133.5342) -> (111.5078, -133.5039)
  line L715 (111.5078, -133.5039) -> (111.5499, -133.4813)
  line L716 (111.5499, -133.4813) -> (111.5957, -133.4676)
  line L717 (111.5957, -133.4676) -> (111.6432, -133.4628)
  line L718 (111.6432, -133.4628) -> (112.1308, -133.4628)
  line L719 (112.1308, -133.4628) -> (112.1783, -133.4676)
  line L720 (108.6061, -133.479) -> (108.6521, -133.493)
  line L721 (108.6521, -133.493) -> (108.694, -133.5154)
  line L722 (108.694, -133.5154) -> (108.7311, -133.5458)
  line L723 (108.7311, -133.5458) -> (108.7613, -133.5827)
  line L724 (108.7613, -133.5827) -> (108.7839, -133.6248)
  line L725 (108.7839, -133.6248) -> (108.7976, -133.6705)
  line L726 (108.7976, -133.6705) -> (108.8024, -133.718)
  line L727 (108.8024, -133.718) -> (108.8024, -134.2057)
  line L728 (108.8024, -134.2057) -> (108.7976, -134.2532)